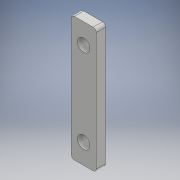
# Autodesk Inventor part: load_cell
Saved by Autodesk Inventor 2018 (Build 220112000, 112)
## iProperties
Created: 2018-12-03
Part Number: load_cell
Material: Generic
Document SubType Name: Modeling
Designer: jaspe
Density: 1 g/cm^3
Appearance: Default
Author: jaspe
Autodesk Inventor part; units mm, degrees
ref_plane "YZ Plane" through (0, 0, 0) normal (1, 0, 0) x (0, 1, 0)
ref_plane "XZ Plane" through (0, 0, 0) normal (0, 1, 0) x (-1, 0, 0)
ref_plane "XY Plane" through (0, 0, 0) normal (0, 0, 1) x (1, 0, 0)
sketch "Sketch1" plane through (0, 0, 0) normal (0, 1, 0) x (-1, 0, 0)
  line L0 (-4, 20) -> (4, 20)
  line L1 (4, 20) -> (4, -20)
  line L2 (4, -20) -> (-4, -20)
  line L3 (-4, -20) -> (-4, 20)
  line L4 (-4, 20) -> (4, -20) construction
  line L5 (4, 20) -> (-4, -20) construction
  point P0 (0, 0)
  dimension "d0" = 8
  dimension "d1" = 40
  constraints: 12 end point, 2 midpoint, 2 parallel, 1 horizontal, 1 perpendicular
  measures "d0" distance of L1.end L2.end
  measures "d1" distance of L0.end L1.end
extrude "Extrusion1" add sketch "Sketch1" along normal blind 3
fillet "Fillet1" radius 1 4 edges at (4, 1.5, 20) (-4, 1.5, 20) (4, 1.5, -20) (-4, 1.5, -20)
sketch "Sketch2" plane through (0, 3, 0) normal (0, 1, 0) x (1, 0, 0)
  line L0 (0, 0) -> (0, -13.5) construction
  line L1 (0, 0) -> (0, 13.5) construction
  circle A0 centre (0, -13.5) radius 2
  circle A1 centre (0, 13.5) radius 2
  dimension "d5" = 13.5
  dimension "d6" = 13.5
  dimension "d7" = 4
  dimension "d8" = 4
  constraints: 4 end point, 2 centre point, 2 coincident, 2 vertical
  measures "d5" distance of L0.start L0.end
  measures "d6" distance of L0.start L1.end
  measures "d7" diameter of A0
  measures "d8" diameter of A1
extrude "Extrusion2" cut sketch "Sketch2" against normal up to surface (3 mm away)
sketch "Sketch3" plane through (0, 3, 0) normal (0, 1, 0) x (1, 0, 0)
  line L0 (-4, 9.5) -> (4, 9.5)
  line L1 (4, 9.5) -> (4, -9.5)
  line L2 (4, -9.5) -> (-4, -9.5)
  line L3 (-4, -9.5) -> (-4, 9.5)
  line L4 (-4, 9.5) -> (4, -9.5) construction
  line L5 (4, 9.5) -> (-4, -9.5) construction
  point P0 (0, 0)
  dimension "d11" = 8
  dimension "d12" = 19
  constraints: 12 end point, 2 midpoint, 2 parallel, 1 horizontal, 1 perpendicular
  measures "d11" distance of L1.end L2.end
  measures "d12" distance between parallel lines of L0 L2
extrude "Extrusion3" add sketch "Sketch3" along normal blind 1
chamfer "Chamfer1" distance 1 angle 45 4 edges at (0, 4, 9.5) (0, 4, -9.5) (4, 4, 0) (-4, 4, 0)
body "Solid1"
